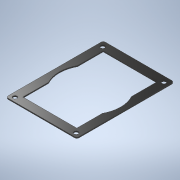
# Autodesk Inventor part: Part1
Saved by Autodesk Inventor 2020.3 (Build 243373000, 373)
## iProperties
Created: 2020-07-15
Part Number: Part1
Material: Generic
Document SubType Name: Modeling
Designer: mifer
Density: 1 g/cm^3
Appearance: Glossy - Black
Author: mifer
Autodesk Inventor part; units mm, degrees
ref_plane "YZ Plane" through (0, 0, 0) normal (1, 0, 0) x (0, 1, 0)
ref_plane "XZ Plane" through (0, 0, 0) normal (0, 1, 0) x (-1, 0, 0)
ref_plane "XY Plane" through (0, 0, 0) normal (0, 0, 1) x (1, 0, 0)
sketch "Sketch1" plane through (0, 0, 0) normal (0, 1, 0) x (-1, 0, 0)
  line L0 (2, 0) -> (65, 0)
  line L1 (67, -2) -> (67, -90)
  line L2 (65, -92) -> (2, -92)
  line L3 (0, -90) -> (0, -2)
  arc A0 (67, -2) -> (65, 0) centre (65, -2) ccw
  arc A1 (65, -92) -> (67, -90) centre (65, -90) ccw
  arc A2 (0, -90) -> (2, -92) centre (2, -90) ccw
  arc A3 (2, 0) -> (0, -2) centre (2, -2) ccw
  line L4 (8, -8) -> (59, -8)
  line L5 (59, -84) -> (8, -84)
  line L6 (59, -8) -> (59, -32.2523)
  line L7 (59, -59.7477) -> (59, -84)
  line L8 (8, -84) -> (8, -59.7477)
  line L9 (8, -32.2523) -> (8, -8)
  arc A4 (59, -59.7477) -> (59, -32.2523) centre (33.5, -46) ccw
  arc A5 (8, -32.2523) -> (8, -59.7477) centre (33.5, -46) ccw
  circle A6 centre (62.4698, -4) radius 2
  circle A7 centre (62.4698, -87) radius 2
  circle A8 centre (4.5302, -4) radius 2
  circle A9 centre (4.5302, -87) radius 2
  point P0 (0, 0)
  point P1 (67, -92)
  point P2 (67, 0)
  point P3 (0, -92)
  dimension "d40" = 67
  dimension "d41" = 92
  dimension "d42" = 2
  dimension "d43" = 51
  dimension "d44" = 76
  constraints: 20 end point, 12 point on circle, 10 centre point, 8 point on line, 8 tangent, 7 parallel, 3 equal radius, 3 perpendicular, 2 horizontal
  measures "d40" distance of point (67, -92) point (0, -92)
  measures "d41" distance of point (67, 0) point (67, -92)
  measures "d42" radius of A0
  measures "d43" distance of L5.start L5.end
  measures "d44" distance of L4.end L5.start
extrude "Extrusion9" add sketch "Sketch1" along normal blind 1
body "Solid5"
